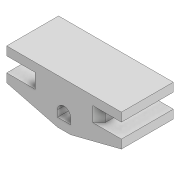
# Autodesk Inventor part: glass_holder
Saved by Autodesk Inventor 2022 (Build 260153000, 153)
## iProperties
Created: 2021-09-02
Part Number: glass_holder
Material: Generic
Document SubType Name: Modeling
Designer: Daniel
Density: 1 g/cm^3
Appearance: Default
Author: Daniel
Autodesk Inventor part; units mm, degrees
ref_plane "YZ Plane" through (0, 0, 0) normal (1, 0, 0) x (0, 1, 0)
ref_plane "XZ Plane" through (0, 0, 0) normal (0, 1, 0) x (-1, 0, 0)
ref_plane "XY Plane" through (0, 0, 0) normal (0, 0, 1) x (1, 0, 0)
sketch "Sketch1" plane through (0, 0, 0) normal (0, 0, 1) x (1, 0, 0)
  line L0 (-6.635, 1.85) -> (6.635, 1.85)
  line L1 (6.635, 1.85) -> (6.635, -1.85)
  line L2 (6.635, -1.85) -> (0.7071, -1.85)
  line L3 (-6.635, -1.85) -> (-6.635, 1.85)
  line L4 (-6.635, 1.85) -> (6.635, -1.85) construction
  line L5 (6.635, 1.85) -> (-6.635, -1.85) construction
  line L6 (-6.635, 0.85) -> (-4.035, 0.85)
  line L7 (-4.035, 0.85) -> (-4.035, -0.85)
  line L8 (-4.035, -0.85) -> (-6.635, -0.85)
  line L9 (-6.635, -0.85) -> (-6.635, 0.85)
  line L10 (6.635, 0.85) -> (4.035, 0.85)
  line L11 (4.035, 0.85) -> (4.035, -0.85)
  line L12 (4.035, -0.85) -> (6.635, -0.85)
  line L13 (6.635, -0.85) -> (6.635, 0.85)
  line L14 (-4.035, 0) -> (-6.635, 0) construction
  line L15 (6.635, 0) -> (4.035, 0) construction
  circle A0 centre (0, -1.6) radius 0.75
  line L16 (-0.75, -2.35) -> (0.75, -2.35)
  line L17 (0.75, -2.35) -> (0.75, -1.85)
  line L18 (-0.75, -2.35) -> (-0.75, -1.85)
  line L19 (-0.7071, -1.85) -> (-6.635, -1.85)
  line L20 (0.7071, -1.85) -> (-0.7071, -1.85)
  line L21 (-6.635, -1.85) -> (-0.75, -3.35)
  line L22 (-0.75, -3.35) -> (0.75, -3.35)
  line L23 (0.75, -3.35) -> (6.635, -1.85)
  line L24 (-0.75, -1.85) -> (-0.75, -1.6)
  line L25 (0.75, -1.85) -> (0.75, -1.6)
  point P0 (0, 0)
  point P1 (0, 0)
  point P2 (0, 0)
  dimension "d0" = 2.6
  dimension "d1" = 2.6
  dimension "d2" = 13.27
  dimension "d3" = 1.7
  dimension "d4" = 1
  dimension "d7" = 1.5
  dimension "d8" = 1
  constraints: 52 end point, 11 parallel, 9 point on line, 8 midpoint, 6 tangent, 4 horizontal, 4 point on circle, 3 perpendicular, 3 vertical, 3 vertical alignment, 1 centre point
  measures "d0" distance between parallel lines of L3 L7
  measures "d1" distance between parallel lines of L1 L11
  measures "d2" distance of L0.start L0.end
  measures "d3" distance between parallel lines of L8 L6
  measures "d4" distance between parallel lines of L0 L6
  measures "d7" diameter of A0
  measures "d8" distance between parallel lines of L16 L22
extrude "Extrusion2" add sketch "Sketch1" along normal blind 6 contours L0 L1 L10 L11 L12 L2 L25 A0 L24 L19 L3 L8 L7 L6 | L19 L18 L16 L17 L2 L23 L22 L21
chamfer "Chamfer1" distance 0.7 angle 45 2 edges at (-4.035, 0, 6) (4.035, 0, 6)
equation "\"d1\" = d0"
body "Solid2"
